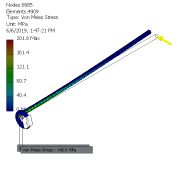
# Autodesk Inventor part: Mono spreader
Saved by Autodesk Inventor 2017 (Build 210142000, 142)
## iProperties
Created: 2019-06-06
Part Number: Mono spreader
Material: Steel
Document SubType Name: Modeling
Designer: Admin
Mass: 179.864 g
Surface Area: 114.648 cm^2
Volume: 22.9126 cm^3
Density: 7.85 g/cm^3
Appearance: Plate
Author: Admin
Autodesk Inventor part; units mm, degrees
ref_plane "YZ Plane" through (0, 0, 0) normal (1, 0, 0) x (0, 1, 0)
ref_plane "XY Plane" through (0, 0, 0) normal (0, 0, 1) x (1, 0, 0)
ref_plane "Work Plane1" through (0, 30, 0) normal (0, 1, 0) x (-1, 0, 0)
sketch "Sketch4" plane through (0, 0, 0) normal (0, 1, 0) x (-1, 0, 0)
  circle A0 centre (0, 0) radius 4
  dimension "d8" = 8
  constraints: 1 centre point, 1 coincident
  measures "d8" diameter of A0
extrude "Extrusion1" add sketch "Sketch4" along normal blind 365
sketch "Sketch5" plane through (0, 0, 0) normal (0, -1, 0) x (1, 0, 0)
  line L0 (0, 0) -> (30, 0)
  circle A0 centre (15, 0) radius 15
  dimension "d11" = 30
  constraints: 2 end point, 1 horizontal, 1 horizontal alignment, 1 midpoint, 2 other
  measures "d11" distance of L0.start L0.end
sketch "Sketch6" plane through (0, 0, 0) normal (0, 0, 1) x (1, 0, 0)
  circle A0 centre (0, 0) radius 4
  line L0 (-4, 0) -> (-4, 365) projected
  constraints: 1 centre point, 1 coincident, 1 tangent
sweep "Sweep2" add profiles "Sketch6" path "Sketch5" path curves A0
body "Solid4"
